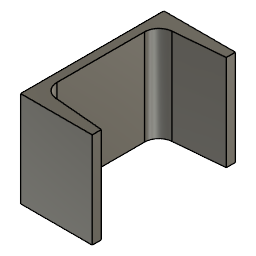
C-150×75×9×12.5 (Autodesk Fusion 360 design; units mm, degrees)
Autodesk Fusion 360 part; units mm, degrees
note: some values were not read from the file. Set by a fixed rule: which sketch regions a step uses.
sketch "スケッチ1" plane through (0, 0, 0) normal (0, 0, 1) x (1, 0, 0)
  line L0 (9, 120.8679) -> (9, 29.1321)
  line L1 (0, 150) -> (0, 0)
  line L2 (0, 0) -> (75, 0)
  line L3 (22.6927, 14.1892) -> (75, 9.6129)
  arc A0 (9, 29.1321) -> (22.6927, 14.1892) centre (24, 29.1321) ccw
  line L4 (75, 9.6129) -> (75, 0)
  line L5 (75, 140.3871) -> (22.6927, 135.8108)
  line L6 (0, 150) -> (75, 150)
  arc A1 (22.6927, 135.8108) -> (9, 120.8679) centre (24, 120.8679) ccw
  line L7 (75, 150) -> (75, 140.3871)
extrude "押し出し1" add sketch "スケッチ1" along normal blind 100
